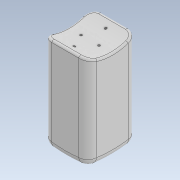
# Autodesk Inventor part: shank_link
Saved by Autodesk Inventor 2020 (Build 240168000, 168)
## iProperties
Created: 2020-12-22
Part Number: shank_link
Material: Generic
Document SubType Name: Modeling
Designer: DELL
Density: 1 g/cm^3
Appearance: Default
Author: DELL
Autodesk Inventor part; units mm, degrees
sketch "Sketch1" plane through (0, 0, 0) normal (1, 0, 0) x (0, 1, 0)
  line L0 (0, 0) -> (0, 25.2399) construction
  line L1 (0, 0) -> (0, -46.7601) construction
  line L2 (0, 0) -> (-130, 0) construction
  circle A0 centre (0, 0) radius 27.5
  line L3 (0, 27.5) -> (-130, 27.5)
  line L4 (0, -27.5) -> (-130, -27.5)
  line L5 (-130, 27.5) -> (-130, -27.5)
  line L6 (0, 0) -> (27.5, 0) construction
  circle A1 centre (0, 0) radius 130 construction
  arc A2 (-127.0581, 27.5) -> (-127.0581, -27.5) centre (0, 0) ccw
  line L7 (0, 0) -> (0, 27.5) construction
  line L8 (0, 0) -> (-130, 0)
  line L9 (-123.6932, 40) -> (-130, 40)
  line L10 (-130, 40) -> (-130, 0)
  arc A3 (-123.6932, 40) -> (-130, 0) centre (0, 0) ccw
  arc A4 (-20.1314, 27.5) -> (-20.1314, -27.5) centre (27.5, 0) ccw
  point P0 (-65, 0)
  point P1 (-130, 0)
  point P2 (-130, 27.5)
  point P3 (-127.0581, 27.5)
  dimension "d6" = 55
  dimension "d84" = 130
  dimension "d85" = 55
  dimension "d129" = 27.5
  dimension "d130" = 127.0581
  dimension "d131" = 2.9419
  dimension "d134" = 40
  dimension "d137" = 110
  constraints: 22 end point, 13 point on circle, 7 point on line, 5 centre point, 5 coincident, 2 collinear, 2 midpoint, 2 perpendicular, 2 tangent, 2 vertical, 1 horizontal, 1 symmetric about line, 1 other
  measures "d6" diameter of A0
  measures "d84" distance between parallel lines of L5 L1
  measures "d85" distance of L3.end L4.end
  measures "d129" distance from line of A1.end L2
  measures "d130" distance from line of L0 A1.end
  measures "d131" distance from line of L5 A1.end
  measures "d134" distance from line of L2.end L9
  measures "d137" diameter of A4
ref_plane "Work Plane1" through (14.5, 0, 0) normal (1, 0, 0) x (0, 1, 0)
ref_plane "Work Plane2" through (20, 0, 0) normal (1, 0, 0) x (0, 1, 0)
extrude "Extrusion4" add sketch "Sketch1" along normal mid plane 50 contours A4 L4 A2 L8 | L8 A2 L3 A4
revolve "Revolution1" cut sketch "Sketch1" angle 360 about axis through (0, 0, 0) along (0, -1, 0) contours L5 L3 A2 | L3 L10 L9 A3
sketch "Sketch6" plane through (0, 0, 0) normal (0, 1, 0) x (-1, 0, 0)
  circle A0 centre (0, 0) radius 10
  line L0 (-25, -27.5) -> (-25, 27.5) projected
  point P0 (-25, 27.5)
  point P1 (0, 0)
  dimension "d123" = 20
  constraints: 2 coincident, 1 centre point, 1 other
  measures "d123" diameter of A0
ref_plane "Work Plane5" through (0, -130, 0) normal (0, 1, 0) x (-1, 0, 0)
extrude "Extrusion11" cut sketch "Sketch6" along normal blind 60 from surface at -130
fillet "Fillet28" radius 10 4 edges at (25, -72.3528, -27.5) (25, -72.3528, 27.5) (-25, -72.3528, 27.5) (-25, -72.3528, -27.5)
fillet "Fillet29" radius 8 7 edges at (25, -127.5735, 0) (0, -127.0581, -27.5) (-22.0799, -125.7345, -24.5622) (-25, -127.5735, 0) (-22.0799, -125.7345, 24.5622) (-7.5131, -126.8357, 27.5) (7.5131, -126.8357, 27.5)
fillet "Fillet36" radius 2 8 edges at (21.6907, -21.5244, 24.932) (0, -20.1314, 27.5) (-21.8817, -21.6138, 24.7555) (-25, -27.5, 0) (-21.6893, -21.5238, -24.9332) (0, -20.1314, -27.5) (21.6893, -21.5238, -24.9332) (25, -27.5, 0)
sketch "Sketch7" plane through (0, 0, 0) normal (0, 1, 0) x (-1, 0, 0)
  circle A0 centre (0, 17.5) radius 1.25
  circle A1 centre (0, -17.5) radius 1.25
  line L0 (-24.8538, 0) -> (25, 0) construction
  line L1 (0, -27.5) -> (0, 28.33) construction
  circle A2 centre (-10, 0) radius 1.25
  circle A3 centre (10, 0) radius 1.25
  line L2 (25, -17.5) -> (25, 17.5) projected
  line L3 (-15, -27.5) -> (15, -27.5) projected
  dimension "d140" = 2.5
  dimension "d142" = 20
  dimension "d143" = 35
  constraints: 4 centre point, 4 end point, 3 equal radius, 3 point on line, 2 midpoint, 2 symmetric about line, 1 horizontal
  measures "d140" diameter of A0
  measures "d142" distance of A3.centre A2.centre
  measures "d143" distance of A0.centre A1.centre
extrude "Extrusion12" cut sketch "Sketch7" against normal blind 40
body "Solid1"
